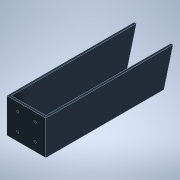
# Autodesk Inventor part: Soporte Cilindro Cortadora
Saved by Autodesk Inventor 2021 (Build 250183000, 183)
## iProperties
Created: 2021-07-14
Part Number: Soporte Cilindro Cortadora
Material: Generic
Document SubType Name: Modeling
Designer: maaro
Density: 1 g/cm^3
Appearance: Default(2)
Author: maaro
Autodesk Inventor part; units mm, degrees
ref_plane "YZ Plane" through (0, 0, 0) normal (1, 0, 0) x (0, 1, 0)
ref_plane "XZ Plane" through (0, 0, 0) normal (0, 1, 0) x (-1, 0, 0)
ref_plane "XY Plane" through (0, 0, 0) normal (0, 0, 1) x (1, 0, 0)
sketch "Sketch1" plane through (0, 0, 0) normal (0, 0, 1) x (1, 0, 0)
  line L0 (-37.5, 37.5) -> (37.5, 37.5)
  line L1 (37.5, 37.5) -> (37.5, -37.5)
  line L2 (37.5, -37.5) -> (-37.5, -37.5)
  line L3 (-37.5, -37.5) -> (-37.5, 37.5)
  line L4 (-37.5, 37.5) -> (37.5, -37.5) construction
  line L5 (37.5, 37.5) -> (-37.5, -37.5) construction
  circle A0 centre (0, 0) radius 37.5 projected
  circle A1 centre (19, -19) radius 2.4585 projected
  circle A2 centre (19, 19) radius 2.4585 projected
  circle A3 centre (-19, 19) radius 2.4585 projected
  circle A4 centre (-19, -19) radius 2.4585 projected
  point P0 (0, 0)
  constraints: 12 end point, 2 midpoint, 2 parallel, 2 tangent, 1 horizontal, 1 perpendicular
extrude "Extrusion1" add sketch "Sketch1" along normal blind 5
sketch "Sketch2" plane through (37.5, -37.5, 0) normal (1, 0, 0) x (0, 0, -1)
  line L0 (25.7498, -847.0546) -> (318.6402, 246.0273) projected
  line L1 (-5, 75) -> (-5, 0) projected
  line L2 (-5, 75) -> (272.8136, 75)
  line L3 (252.7174, 0) -> (-5, 0)
  point P0 (0, 37.5)
  constraints: 4 end point, 2 horizontal, 2 point on line
extrude "Extrusion2" add sketch "Sketch2" along normal blind 5
mirror "Mirror1" about plane through (0, 0, 0) normal (1, 0, 0) of "Extrusion2"
body "Solid1"
